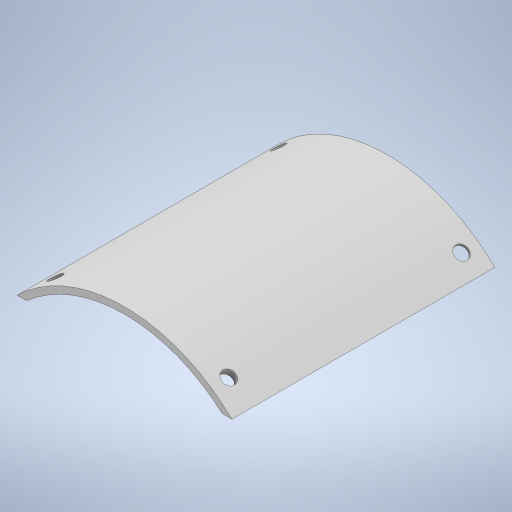
# Autodesk Inventor part: Electronics Door
Saved by Autodesk Inventor 2024 (Build 280153000, 153)
## iProperties
Created: 2024-04-23
Part Number: Electronics Door
Material: Generic
Document SubType Name: Modeling
Designer: auror
Density: 1 g/cm^3
Appearance: Default
Author: auror
Autodesk Inventor part; units mm, degrees
ref_plane "YZ Plane" through (0, 0, 0) normal (1, 0, 0) x (0, 1, 0)
ref_plane "XZ Plane" through (0, 0, 0) normal (0, 1, 0) x (-1, 0, 0)
ref_plane "XY Plane" through (0, 0, 0) normal (0, 0, 1) x (1, 0, 0)
sketch "Sketch8" plane through (0, 0, 0) normal (0, 0, 1) x (1, 0, 0)
  arc A0 (23.7678, 25.0068) -> (-23.7678, 25.0068) centre (0, 0) ccw
  arc A1 (24.495, 24.9999) -> (-24.495, 24.9999) centre (0, 0) ccw
  line L0 (-23.7678, 25.0068) -> (-24.495, 24.9999)
  line L1 (-24.6461, 24.172) -> (-22.9143, 25.818) construction
  line L2 (22.991, 25.7452) -> (24.5566, 24.2571) construction
  line L3 (23.7678, 25.0068) -> (24.495, 24.9999)
  line L4 (-24.495, 24.9999) -> (24.495, 24.9999) construction
  dimension "d88" = 34.5
  dimension "d89" = 35
  dimension "d90" = 0
  dimension "d91" = 137
  dimension "d92" = 0
  dimension "d93" = 137
  dimension "d98" = 48.99
  constraints: 10 end point, 4 point on circle, 2 centre point, 2 coincident, 2 tangent, 1 horizontal
  measures "d88" radius of A0
  measures "d89" radius of A1
  measures "d90" distance from line of L0.start L1
  measures "d91" angle of L0 L1
  measures "d92" distance from line of L3.start L2
  measures "d93" angle of L3 L2
  measures "d98" distance of L0.end L3.end
extrude "Extrusion5" add sketch "Sketch8" along normal blind 60
sketch "Sketch9" plane through (0, 0, 60) normal (0, 0, 1) x (1, 0, 0)
  arc A0 (22.2755, 25.021) -> (-22.2755, 25.021) centre (0, 0) ccw
  arc A1 (23.7678, 25.0068) -> (-23.7678, 25.0068) centre (0, 0) ccw projected
  line L0 (-23.7678, 25.0068) -> (-22.2755, 25.021)
  line L1 (-24.495, 24.9999) -> (-23.7678, 25.0068) projected
  line L2 (23.7678, 25.0068) -> (22.2755, 25.021)
  line L3 (23.7678, 25.0068) -> (24.495, 24.9999) projected
  dimension "d96" = 33.5
  constraints: 4 end point, 2 collinear, 2 point on circle, 1 centre point, 1 coincident
  measures "d96" radius of A0
extrude "Extrusion6" add sketch "Sketch9" against normal blind 12.5
sketch "Sketch19" plane through (0, 0, 60) normal (0, 0, 1) x (1, 0, 0)
  line L0 (-24.495, 24.9999) -> (-22.2755, 25.021) construction
  line L1 (-22.2755, 25.021) -> (-7.4699, 32.6566) construction
  arc A0 (22.2755, 25.021) -> (-22.2755, 25.021) centre (0, 0) ccw construction
  dimension "d162" = 32.448
  constraints: 2 end point, 1 point on circle
  measures "d162" distance from line of point (0, 0) L1
sketch "Sketch20" plane through (0, 0, 0) normal (0, 0, -1) x (-1, 0, 0)
  arc A0 (22.2755, 25.021) -> (-22.2755, 25.021) centre (0, 0) ccw projected
  line L0 (22.2755, 25.021) -> (7.4699, 32.6566) construction
  dimension "d163" = 32.448
  constraints: 2 end point, 1 point on circle
  measures "d163" distance from line of point (0, 0) L0
ref_plane "Work Plane10" through (-22.2755, 25.021, 0) normal (0.458355, -0.8887692, 0) x (0.8887692, 0.458355, 0)
sketch "Sketch21" plane through (-22.2755, 25.021, 0) normal (0.458355, -0.8887692, 0) x (0.8887692, 0.458355, 0)
  line L0 (-1.3328, 0) -> (40.9154, 0) projected
  line L1 (0, 60) -> (39.5956, 60) projected
  line L2 (0, 60) -> (0, 47.5) projected
  line L3 (-1.3328, 0) -> (-1.3328, 47.5) projected
  point P0 (8.3293, 0)
  point P1 (2.6672, 4)
  point P2 (4, 56)
  dimension "d164" = 4
  dimension "d165" = 4
  dimension "d166" = 4
  dimension "d167" = 4
  measures "d164" distance from line of L0 point (2.667, 4)
  measures "d165" distance from line of L1 point (4, 56)
  measures "d166" distance from line of point (4, 56) L2
  measures "d167" distance from line of L3 point (2.667, 4)
hole "Hole10" at (-19.905, 26.2435, 4) at (-18.7205, 26.8544, 56) direction (-0.458355, 0.8887692, 0) diameter 3.1 end through all
ref_plane "Work Plane11" through (0, 25.2328, 0) normal (1, 0, 0) x (0, 0, 1)
mirror "Mirror1" about plane through (0, 25.2328, 0) normal (1, 0, 0) of "Hole10"
body "Solid2"
